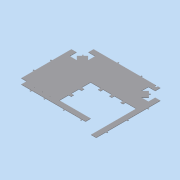
# Autodesk Inventor part: rx_v1_23_cu_shield_no-folds
Saved by Autodesk Inventor 2014 (Build 180170000, 170)
## iProperties
Created: 2013-10-31
Part Number: rx_v1_23_cu_shield_no-folds
Material: Generic
Document SubType Name: Sheet Metal
Designer: Robert Davis
Density: 1 g/cm^3
Sheet Metal Rule: Default_mm
Flat Pattern Width: 10.6083 cm
Flat Pattern Length: 8.8649 cm
Flat Pattern Area: 94.0415 cm^2
Sheet Metal Width: 106.083 mm
Sheet Metal Length: 88.649 mm
Sheet Metal Area: 9404.152 mm^2
Appearance: Default
Author: Robert Davis
Autodesk Inventor part; units mm, degrees
ref_plane "YZ Plane" through (0, 0, 0) normal (1, 0, 0) x (0, 1, 0)
ref_plane "XZ Plane" through (0, 0, 0) normal (0, 1, 0) x (-1, 0, 0)
ref_plane "XY Plane" through (0, 0, 0) normal (0, 0, 1) x (1, 0, 0)
ref_plane "Work Plane21" through (15.9995, 53.041, 0) normal (1, 0, 0) x (0, 1, 0)
ref_plane "Work Plane22" through (-11.0005, 53.041, 0) normal (1, 0, 0) x (0, 1, 0)
sketch "Sketch1" plane through (0, 0, 0) normal (0, 0, 1) x (1, 0, 0)
  line L0 (0, 0) -> (0, 10)
  line L1 (-38.7075, 51.541) -> (-38.7075, 45.574)
  line L2 (-38.7075, 45.574) -> (-30.8075, 45.574)
  line L3 (-30.8075, 45.574) -> (-30.8075, 37.3477)
  line L4 (-30.8075, 37.3477) -> (-35.2149, 41.7551)
  line L5 (-41.7556, 35.2144) -> (-37.3482, 30.807)
  line L6 (-37.3482, 30.807) -> (-45.5745, 30.807)
  line L7 (-45.5745, 30.807) -> (-45.5745, 38.707)
  line L8 (-45.5745, 38.707) -> (-51.5415, 38.707)
  line L9 (38.7075, 51.541) -> (38.7075, 45.574)
  line L10 (38.7075, 45.574) -> (30.8075, 45.574)
  line L11 (30.8075, 45.574) -> (30.8075, 37.3477)
  line L12 (30.8075, 37.3477) -> (35.2149, 41.7551)
  line L13 (41.7556, 35.2144) -> (37.3482, 30.807)
  line L14 (37.3482, 30.807) -> (45.5745, 30.807)
  line L15 (45.5745, 30.807) -> (45.5745, 38.707)
  line L16 (45.5745, 38.707) -> (51.5415, 38.707)
  line L17 (-51.5415, -19.309) -> (-45.3065, -19.309)
  line L18 (-45.3065, -19.309) -> (-45.3065, -25.544)
  line L19 (29.1075, -25.544) -> (29.1075, -19.577)
  line L20 (29.1075, -19.577) -> (-7.1925, -19.577)
  line L21 (45.5745, 16.692) -> (45.5745, -35.608)
  line L22 (45.5745, -35.608) -> (51.5415, -35.608)
  line L23 (-11.5005, 53.041) -> (-10.5005, 53.041)
  line L24 (-10.5005, 53.041) -> (-10.5005, 51.541)
  line L25 (-11.5005, 51.541) -> (-11.5005, 53.041)
  line L26 (15.4995, 53.041) -> (16.4995, 53.041)
  line L27 (16.4995, 53.041) -> (16.4995, 51.541)
  line L28 (15.4995, 51.541) -> (15.4995, 53.041)
  line L29 (15.4995, 51.541) -> (-10.5005, 51.541)
  line L30 (-11.5005, 51.541) -> (-38.7075, 51.541)
  line L31 (-51.5415, 16.499) -> (-53.0415, 16.499)
  line L32 (-53.0415, 16.499) -> (-53.0415, 15.499)
  line L33 (-53.0415, 15.499) -> (-51.5415, 15.499)
  line L34 (-51.5415, -3.501) -> (-53.0415, -3.501)
  line L35 (-53.0415, -3.501) -> (-53.0415, -4.501)
  line L36 (-53.0415, -4.501) -> (-51.5415, -4.501)
  line L37 (-51.5415, 38.707) -> (-51.5415, 16.499)
  line L38 (-51.5415, 15.499) -> (-51.5415, -3.501)
  line L39 (-51.5415, -4.501) -> (-51.5415, -19.309)
  line L40 (-38.609, 38.361) -> (-39.6697, 39.4217)
  line L41 (-39.6697, 39.4217) -> (-38.9626, 40.1288)
  line L42 (-38.9626, 40.1288) -> (-37.9019, 39.0681)
  line L43 (-35.2149, 41.7551) -> (-37.9019, 39.0681)
  line L44 (-38.609, 38.361) -> (-41.7556, 35.2144)
  line L45 (37.9019, 39.0681) -> (38.9626, 40.1288)
  line L46 (38.9626, 40.1288) -> (39.6697, 39.4217)
  line L47 (39.6697, 39.4217) -> (38.609, 38.361)
  line L48 (35.2149, 41.7551) -> (37.9019, 39.0681)
  line L49 (38.609, 38.361) -> (41.7556, 35.2144)
  line L50 (51.5415, 24.119) -> (53.0415, 24.119)
  line L51 (53.0415, 24.119) -> (53.0415, 23.119)
  line L52 (53.0415, 23.119) -> (51.5415, 23.119)
  line L53 (51.5415, 0.618) -> (53.0415, 0.618)
  line L54 (53.0415, 0.618) -> (53.0415, -0.382)
  line L55 (53.0415, -0.382) -> (51.5415, -0.382)
  line L56 (51.5415, -23.382) -> (53.0415, -23.382)
  line L57 (53.0415, -23.382) -> (53.0415, -24.382)
  line L58 (53.0415, -24.382) -> (51.5415, -24.382)
  line L59 (51.5415, -24.382) -> (51.5415, -35.608)
  line L60 (51.5415, -0.382) -> (51.5415, -23.382)
  line L61 (51.5415, 38.707) -> (51.5415, 24.119)
  line L62 (51.5415, 23.119) -> (51.5415, 0.618)
  line L63 (-34.0005, -25.544) -> (-34.0005, -27.044)
  line L64 (-34.0005, -27.044) -> (-33.0005, -27.044)
  line L65 (-33.0005, -27.044) -> (-33.0001, -25.544)
  line L66 (-17.0001, -25.544) -> (-17.0005, -27.044)
  line L67 (-17.0005, -27.044) -> (-18.0005, -27.044)
  line L68 (-18.0005, -27.044) -> (-18.0005, -25.544)
  line L69 (5.3815, -25.544) -> (5.3815, -27.044)
  line L70 (5.3815, -27.044) -> (4.3815, -27.044)
  line L71 (4.3815, -27.044) -> (4.3815, -25.544)
  line L72 (25.3815, -25.544) -> (25.3815, -27.044)
  line L73 (25.3815, -27.044) -> (24.3815, -27.044)
  line L74 (24.3815, -27.044) -> (24.3815, -25.544)
  line L75 (-45.3065, -25.544) -> (-34.0005, -25.544)
  line L76 (-33.0001, -25.544) -> (-18.0005, -25.544)
  line L77 (-17.0001, -25.544) -> (4.3815, -25.544)
  line L78 (5.3815, -25.544) -> (24.3815, -25.544)
  line L79 (25.3815, -25.544) -> (29.1075, -25.544)
  line L80 (-7.1925, 6.192) -> (-4.1925, 6.192)
  line L81 (-4.1925, 6.192) -> (-4.1925, 3.192)
  line L82 (-4.1925, 3.192) -> (-7.1925, 3.192)
  line L83 (-7.1925, -5.808) -> (-4.1925, -5.808)
  line L84 (-4.1925, -5.808) -> (-4.1925, -8.808)
  line L85 (-4.1925, -8.808) -> (-7.1925, -8.808)
  line L86 (7.3075, 16.692) -> (7.3075, 13.692)
  line L87 (7.3075, 13.692) -> (4.3075, 13.692)
  line L88 (4.3075, 13.692) -> (4.3075, 16.692)
  line L89 (20.3075, 16.692) -> (20.3075, 13.692)
  line L90 (20.3075, 13.692) -> (17.3075, 13.692)
  line L91 (17.3075, 13.692) -> (17.3075, 16.692)
  line L92 (33.3075, 16.692) -> (33.3075, 13.692)
  line L93 (33.3075, 13.692) -> (30.3075, 13.692)
  line L94 (30.3075, 13.692) -> (30.3075, 16.692)
  line L95 (33.3075, 16.692) -> (45.5745, 16.692)
  line L96 (20.3075, 16.692) -> (30.3075, 16.692)
  line L97 (-7.1925, 16.692) -> (4.3075, 16.692)
  line L98 (7.3075, 16.692) -> (17.3075, 16.692)
  line L99 (-7.1925, 6.192) -> (-7.1925, 16.692)
  line L100 (-7.1925, -19.577) -> (-7.1925, -8.808)
  line L101 (-7.1925, -5.808) -> (-7.1925, 3.192)
  arc A0 (33.8055, 50.541) -> (35.8055, 50.541) centre (34.8055, 50.541) ccw
  line L102 (35.8055, 50.541) -> (35.8055, 51.541)
  line L103 (33.8055, 51.541) -> (33.8055, 50.541)
  line L104 (38.7075, 51.541) -> (35.8055, 51.541)
  line L105 (33.8055, 51.541) -> (16.4995, 51.541)
  circle A1 centre (-34.4925, -21.077) radius 0.25
  circle A2 centre (-25.4925, -21.077) radius 0.25
  circle A3 centre (-16.4925, -21.077) radius 0.25
  dimension "d0" = 45
  dimension "d2" = 9.25
  dimension "d3" = 6.233
  dimension "d4" = 7.9
  dimension "d6" = 5.967
  dimension "d8" = 50.116
  dimension "d10" = 36.269
  dimension "d11" = 36.3
  dimension "d13" = 52.3
  dimension "d18" = 1.5
  dimension "d20" = 14.308
  dimension "d22" = 14.808
  dimension "d23" = 1
  dimension "d24" = 9.25
  dimension "d25" = 4.45
  dimension "d27" = 10
  dimension "d34" = 11.306
  dimension "d37" = 3
  dimension "d38" = 3
  dimension "d39" = 11.5
  dimension "d40" = 24.5
  dimension "d41" = 37.5
  dimension "d42" = 10.5
  dimension "d44" = 38.114
  dimension "d46" = 11.574
  dimension "d100" = 6.235
  dimension "d115" = 5.967
  dimension "d159" = 1
  dimension "d161" = 3.998
  dimension "d162" = 1
  dimension "d163" = 9
  dimension "d164" = 9
  dimension "d166" = 0.5
  dimension "d167" = 1.5
  dimension "d168" = 9.3
  dimension "d169" = 20
  dimension "d170" = 16.074
  dimension "d171" = 24
  dimension "d172" = 16
  dimension "d173" = 9
  dimension "d174" = 103.083
  dimension "d175" = 4.45
  dimension "d176" = 27
  dimension "d177" = 20
  dimension "d178" = 14.588
  dimension "d179" = 51.541
  dimension "d180" = 14.767
  measures "d0" angle of L11 L12
  measures "d2" distance of L12.end L13.start
  measures "d3" distance of L3.end L4.end
  measures "d4" distance of L1.end L2.end
  measures "d6" distance of L1.start L1.end
  measures "d8" distance between parallel lines of L17 L6
  measures "d10" distance of L20.end L97.start
  measures "d11" distance of L19.end L20.end
  measures "d13" distance of L21.start L21.end
  measures "d18" distance of L25.start L23.start
  measures "d20" distance between parallel lines of L11 L27
  measures "d22" distance between parallel lines of L36 L17
  measures "d23" distance of L23.start L23.end
  measures "d24" distance between parallel lines of L4 L5
  measures "d25" distance of L40.start L5.start
  measures "d27" distance of L0.start L0.end
  measures "d34" distance between parallel lines of L63 L18
  measures "d37" distance of L92.end L93.end
  measures "d38" distance of L92.start L92.end
  measures "d39" distance between parallel lines of L88 L99
  measures "d40" distance between parallel lines of L91 L99
  measures "d41" distance between parallel lines of L94 L99
  measures "d42" distance of L80.start L97.start
  measures "d44" distance between parallel lines of L100 L18
  measures "d46" distance between parallel lines of L71 L100
  measures "d100" distance of L17.start L17.end
  measures "d115" distance of L19.start L19.end
  measures "d159" radius of A0
  measures "d161" distance from line of L11 A0.centre
  measures "d162" distance from line of L104 A0.centre
  measures "d163" distance of A2.centre A1.centre
  measures "d164" distance of A3.centre A2.centre
  measures "d166" diameter of A2
  measures "d167" distance from line of L20 A2.centre
  measures "d168" distance from line of A3.centre L100
  measures "d169" distance between parallel lines of L72 L69
  measures "d170" distance between parallel lines of L95 L53
  measures "d171" distance between parallel lines of L58 L55
  measures "d172" distance between parallel lines of L66 L65
  measures "d173" distance between parallel lines of L83 L82
  measures "d174" distance between parallel lines of L61 L37
  measures "d175" distance of L47.end L13.start
  measures "d176" distance between parallel lines of L27 L24
  measures "d177" distance between parallel lines of L31 L34
  measures "d178" distance of L16.end L50.start
  measures "d179" distance from line of L30 point (0, 0)
  measures "d180" distance between parallel lines of L3 L7
extrude "Plate1" add sketch "Sketch1" along normal blind 0.381
sketch "Sketch5" plane through (0, 0, 0) normal (0, 0, -1) x (-1, 0, 0)
  line L0 (30.8075, 37.3477) -> (37.3482, 30.807)
  point P0 (0, 0)
  constraints: 2 end point
feature "Fold1" [suppressed]
sketch "Sketch6" plane through (0, 0, 0) normal (0, 0, -1) x (-1, 0, 0)
  line L0 (-30.8075, 37.3477) -> (-37.3482, 30.807)
  point P0 (0, 0)
  constraints: 2 end point
feature "Fold2" [suppressed]
sketch "Sketch8" plane through (0, 0, 0) normal (0, 0, -1) x (-1, 0, 0)
  line L0 (-38.7075, 51.541) -> (-16.4995, 51.541) projected
  line L1 (-30.8075, 45.574) -> (-38.7075, 45.574) projected
  line L2 (-30.8075, 37.3477) -> (-30.8075, 45.574) projected
  line L3 (-30.8085, 45.574) -> (-30.8085, 51.541)
  point P0 (0, 0)
  dimension "d65" = 0.001
  constraints: 2 end point, 2 point on line, 1 perpendicular
  measures "d65" distance between parallel lines of L3 L2
feature "Fold4" [suppressed]
sketch "Sketch9" plane through (0, 0, 0) normal (0, 0, -1) x (-1, 0, 0)
  line L0 (30.8075, 45.574) -> (30.8075, 37.3477) projected
  line L1 (38.7075, 45.574) -> (30.8075, 45.574) projected
  line L2 (11.5005, 51.541) -> (38.7075, 51.541) projected
  line L3 (30.8085, 45.574) -> (30.8085, 51.541)
  point P0 (0, 0)
  dimension "d72" = 0.001
  constraints: 2 end point, 2 point on line, 1 perpendicular
  measures "d72" distance between parallel lines of L0 L3
feature "Fold5" [suppressed]
sketch "Sketch10" plane through (0, 0, 0) normal (0, 0, -1) x (-1, 0, 0)
  line L0 (11.5005, 51.541) -> (38.7075, 51.541) projected
  line L1 (-30.8075, 37.3477) -> (-30.8075, 45.574) projected
  line L2 (30.8075, 45.574) -> (30.8075, 37.3477) projected
  line L3 (-30.8075, 45.573) -> (30.8075, 45.573)
  point P0 (30.8085, 51.541)
  point P1 (0, 0)
  dimension "d79" = 5.968
  constraints: 2 end point, 2 point on line, 1 perpendicular
  measures "d79" distance between parallel lines of L3 L0
feature "Fold6" [suppressed]
sketch "Sketch12" plane through (0, 0, 0) normal (0, 0, -1) x (-1, 0, 0)
  line L0 (51.5415, 38.707) -> (51.5415, 16.499) projected
  line L1 (45.5745, 30.807) -> (45.5745, 38.707) projected
  line L2 (37.3482, 30.807) -> (45.5745, 30.807) projected
  line L3 (45.5745, 30.808) -> (51.5415, 30.808)
  point P0 (0, 0)
  dimension "d92" = 0.001
  constraints: 2 end point, 2 point on line, 1 perpendicular
  measures "d92" distance between parallel lines of L2 L3
feature "Fold8" [suppressed]
sketch "Sketch13" plane through (0, 0, 0) normal (0, 0, -1) x (-1, 0, 0)
  line L0 (37.3482, 30.807) -> (45.5745, 30.807) projected
  line L1 (51.5415, -19.309) -> (45.3065, -19.309) projected
  line L2 (51.5415, 38.707) -> (51.5415, 16.499) projected
  line L3 (45.3085, 30.807) -> (45.3085, -19.309)
  point P0 (51.5415, 30.808)
  point P1 (0, 0)
  dimension "d99" = 6.233
  constraints: 2 end point, 2 point on line, 1 perpendicular
  measures "d99" distance between parallel lines of L2 L3
feature "Fold9" [suppressed]
sketch "Sketch14" plane through (0, 0, 0) normal (0, 0, -1) x (-1, 0, 0)
  line L0 (7.1925, -19.577) -> (7.1925, -8.808) projected
  line L1 (-29.1075, -19.577) -> (7.1925, -19.577) projected
  line L2 (17.0001, -25.544) -> (-4.3815, -25.544) projected
  line L3 (7.1915, -19.577) -> (7.1915, -25.544)
  point P0 (0, 0)
  dimension "d107" = 0.001
  constraints: 2 end point, 2 point on line, 1 perpendicular
  measures "d107" distance between parallel lines of L0 L3
feature "Fold10" [suppressed]
sketch "Sketch15" plane through (0, 0, 0) normal (0, 0, -1) x (-1, 0, 0)
  line L0 (45.3065, -25.544) -> (34.0005, -25.544) projected
  line L1 (45.3065, -19.309) -> (45.3065, -25.544) projected
  line L2 (7.1925, -19.577) -> (7.1925, -8.808) projected
  line L3 (45.3065, -19.309) -> (7.1925, -19.309)
  line L4 (45.3065, -25.544) -> (45.3065, -19.309) projected
  point P0 (0, 0)
  dimension "d114" = 6.235
  constraints: 2 end point, 2 point on line, 1 perpendicular
  measures "d114" distance between parallel lines of L0 L3
feature "Fold11" [suppressed]
sketch "Sketch16" plane through (0, 0, 0) normal (0, 0, -1) x (-1, 0, 0)
  line L0 (-45.5745, 30.807) -> (-37.3482, 30.807) projected
  line L1 (-45.5745, 38.707) -> (-45.5745, 30.807) projected
  line L2 (-51.5415, 24.119) -> (-51.5415, 38.707) projected
  line L3 (-45.5745, 30.808) -> (-51.5415, 30.808)
  point P0 (0, 0)
  dimension "d122" = 0.001
  constraints: 2 end point, 2 point on line, 1 perpendicular
  measures "d122" distance between parallel lines of L0 L3
feature "Fold12" [suppressed]
sketch "Sketch17" plane through (0, 0, 0) normal (0, 0, -1) x (-1, 0, 0)
  line L0 (-51.5415, 0.618) -> (-51.5415, 23.119) projected
  line L1 (-45.5745, 16.692) -> (-45.5745, -35.608) projected
  line L2 (-33.3075, 16.692) -> (-45.5745, 16.692) projected
  line L3 (-45.5745, 16.691) -> (-51.5415, 16.691)
  point P0 (0, 0)
  dimension "d129" = 0.001
  constraints: 2 end point, 2 point on line, 1 perpendicular
  measures "d129" distance between parallel lines of L2 L3
feature "Fold13" [suppressed]
sketch "Sketch18" plane through (0, 0, 0) normal (0, 0, -1) x (-1, 0, 0)
  line L0 (-45.5745, 16.692) -> (-45.5745, -35.608) projected
  line L1 (-33.3075, 16.692) -> (-45.5745, 16.692) projected
  line L2 (-45.5745, 30.807) -> (-37.3482, 30.807) projected
  line L3 (-45.5735, 30.807) -> (-45.5735, 16.692)
  point P0 (-45.5745, 16.691)
  point P1 (0, 0)
  dimension "d136" = 0.001
  constraints: 2 end point, 2 point on line, 1 perpendicular
  measures "d136" distance between parallel lines of L0 L3
feature "Fold14" [suppressed]
sketch "Sketch19" plane through (0, 0, 0) normal (0, 0, -1) x (-1, 0, 0)
  line L0 (4.1925, 6.192) -> (7.1925, 6.192) projected
  line L1 (7.1925, -5.808) -> (7.1925, 3.192) projected
  line L2 (7.1925, -8.808) -> (4.1925, -8.808) projected
  line L3 (6.8105, -8.808) -> (6.8105, 6.192)
  point P0 (0, 0)
  dimension "d143" = 0.382
  constraints: 2 end point, 2 point on line, 1 perpendicular
  measures "d143" distance between parallel lines of L1 L3
feature "Fold15" [suppressed]
sketch "Sketch20" plane through (0, 0, 0) normal (0, 0, -1) x (-1, 0, 0)
  line L0 (-33.3075, 13.692) -> (-33.3075, 16.692) projected
  line L1 (-20.3075, 16.692) -> (-30.3075, 16.692) projected
  line L2 (-4.3075, 16.692) -> (-4.3075, 13.692) projected
  line L3 (-4.3075, 16.31) -> (-33.3075, 16.31)
  point P0 (0, 0)
  dimension "d150" = 0.382
  constraints: 2 end point, 2 point on line, 1 perpendicular
  measures "d150" distance between parallel lines of L1 L3
feature "Fold16" [suppressed]
ref_plane "Work Plane1" through (-45.3065, -25.544, 0.1905) normal (0, 0, 1) x (1, 0, 0)
ref_plane "Work Plane2" through (-33.5005, -27.044, 0.381) normal (-1, 0, 0) x (0, 1, 0)
ref_plane "Work Plane3" through (-17.5005, -27.044, 0.381) normal (-1, 0, 0) x (0, 1, 0)
ref_plane "Work Plane4" through (-51.5415, -19.309, 0.1905) normal (0, 0, 1) x (1, 0, 0)
ref_plane "Work Plane6" through (-53.0415, -4.001, 0.381) normal (0, -1, 0) x (0, 0, -1)
ref_plane "Work Plane7" through (-53.0415, 15.999, 0.381) normal (0, -1, 0) x (0, 0, -1)
ref_plane "Work Plane8" through (29.1075, -25.544, 0.1905) normal (0, 0, 1) x (0, -1, 0)
ref_plane "Work Plane9" through (4.8815, -27.044, 0.381) normal (-1, 0, 0) x (0, 0, 1)
ref_plane "Work Plane10" through (24.8815, -27.044, 0.381) normal (-1, 0, 0) x (0, 0, 1)
ref_plane "Work Plane11" through (51.5415, -35.608, 0.1905) normal (0, 0, 1) x (0, 1, 0)
ref_plane "Work Plane12" through (53.0415, -23.882, 0.381) normal (0, 1, 0) x (1, 0, 0)
ref_plane "Work Plane13" through (53.0415, 0.118, 0.381) normal (0, 1, 0) x (1, 0, 0)
ref_plane "Work Plane14" through (53.0415, 23.119, 0.1905) normal (0, 0, 1) x (1, 0, 0)
ref_plane "Work Plane15" through (53.0415, 23.619, 0.381) normal (0, -1, 0) x (0, 0, 1)
ref_plane "Work Plane16" through (39.6697, 39.4217, 0.1905) normal (0, 0, 1) x (-0.7071068, 0.7071068, 0)
ref_plane "Work Plane17" through (39.3161, 39.7752, 0.381) normal (0.7071068, -0.7071068, 0) x (0, 0, -1)
ref_plane "Work Plane18" through (-39.6697, 39.4217, 0.1905) normal (0, 0, -1) x (-0.7071068, -0.7071068, 0)
ref_plane "Work Plane19" through (-39.3161, 39.7752, 0) normal (-0.7071068, -0.7071068, 0) x (0, 0, 1)
ref_plane "Work Plane20" through (16.4995, 53.041, 0.1905) normal (0, 0, -1) x (1, 0, 0)
equation "\"BendReliefWidth\" = Thickness"
equation "\"BendReliefDepth\" = 0.5 * Thickness"
equation "\"CornerReliefSize\" = 4 * Thickness"
equation "\"MinimumRemnant\" = 2 * Thickness"
equation "\"TransitionRadius\" = BendRadius"
equation "\"JacobiRadiusSize\" = BendRadius"
equation "\"GapSize\" = Thickness"
equation "\"d14\" = BendRadius"
equation "\"Thickness\" = 0.381"
equation "\"BendRadius\" = 0.001"
body "Solid1"
